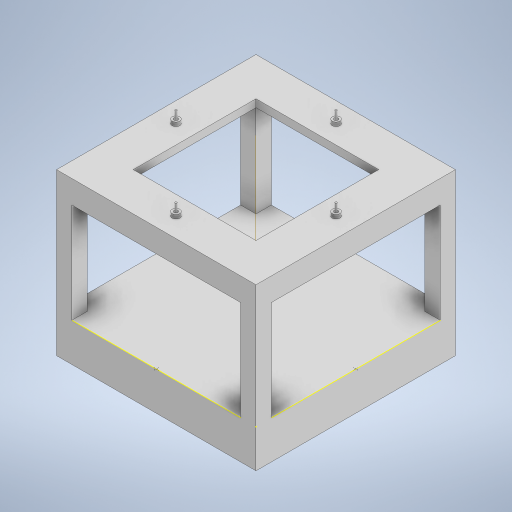
# Autodesk Inventor part: BaseMk1
Saved by Autodesk Inventor 2023 (Build 270158000, 158)
## iProperties
Created: 2023-03-23
Part Number: BaseMk1
Material: Generic
Document SubType Name: Modeling
Designer: czapa
Density: 1 g/cm^3
Appearance: Default
Author: czapa
Autodesk Inventor part; units mm, degrees
ref_plane "YZ Plane" through (0, 0, 0) normal (1, 0, 0) x (0, 1, 0)
ref_plane "XZ Plane" through (0, 0, 0) normal (0, 1, 0) x (-1, 0, 0)
sketch "Sketch1" plane through (0, 0, 0) normal (0, 1, 0) x (-1, 0, 0)
  line L0 (0, 0) -> (260, 0)
  line L1 (260, 0) -> (260, -260)
  line L2 (260, -260) -> (0, -260)
  line L3 (0, -260) -> (0, 0)
  dimension "d0" = 260
  dimension "d1" = 260
  constraints: 8 end point, 2 parallel, 1 horizontal, 1 perpendicular
  measures "d0" distance of L1.end L2.end
  measures "d1" distance of L0.end L1.end
extrude "Extrusion1" add sketch "Sketch1" along normal blind 200
sketch "Sketch2" plane through (0, 200, 0) normal (0, 1, 0) x (1, 0, 0)
  line L0 (-260, 0) -> (0, 0) projected
  line L1 (0, 0) -> (-20, 0)
  line L2 (-20, 0) -> (-20, 20)
  line L3 (-20, 20) -> (0, 20)
  line L4 (0, 20) -> (0, 0)
  line L5 (-260, 260) -> (-260, 0) projected
  line L6 (-260, 260) -> (-240, 260)
  line L7 (-240, 260) -> (-240, 240)
  line L8 (-240, 240) -> (-260, 240)
  line L9 (-260, 240) -> (-260, 260)
  line L10 (-240, 240) -> (-20, 240)
  line L11 (-20, 240) -> (-20, 20)
  line L12 (-20, 20) -> (-240, 20)
  line L13 (-240, 20) -> (-240, 240)
  dimension "d4" = 20
  dimension "d5" = 20
  dimension "d6" = 20
  dimension "d7" = 20
  constraints: 24 end point, 6 parallel, 3 horizontal, 3 perpendicular
  measures "d4" distance of L2.end L3.end
  measures "d5" distance of L1.end L2.end
  measures "d6" distance of L7.end L8.end
  measures "d7" distance of L6.end L7.end
sketch "Sketch3" plane through (-260, 0, 0) normal (0, 0, 1) x (1, 0, 0)
  line L0 (260, 200) -> (0, 200) projected
  line L1 (0, 200) -> (20, 200)
  line L2 (20, 200) -> (20, 180)
  line L3 (20, 180) -> (0, 180)
  line L4 (0, 180) -> (0, 200)
  line L5 (260, 0) -> (240, 0)
  line L6 (240, 0) -> (240, 50)
  line L7 (240, 50) -> (260, 50)
  line L8 (260, 50) -> (260, 0)
  line L9 (20, 180) -> (240, 180)
  line L10 (240, 180) -> (240, 50)
  line L11 (240, 50) -> (20, 50)
  line L12 (20, 50) -> (20, 180)
  dimension "d8" = 20
  dimension "d9" = 20
  dimension "d10" = 20
  dimension "d11" = 50
  constraints: 24 end point, 6 parallel, 3 horizontal, 3 perpendicular
  measures "d8" distance of L2.end L3.end
  measures "d9" distance of L1.end L2.end
  measures "d10" distance of L6.end L7.end
  measures "d11" distance of L5.end L6.end
extrude "Extrusion2" cut sketch "Sketch2" against normal blind 150 contours L12 L13 L10 L11
extrude "Extrusion3" cut sketch "Sketch3" against normal blind 260 contours L9 L10 L11 L12
ref_plane "Work Plane1" through (0, 0, -130) normal (0, 0, 1) x (1, 0, 0)
sketch "Sketch4" plane through (0, 0, 0) normal (1, 0, 0) x (0, 0, -1)
  line L0 (260, 200) -> (0, 200)
  line L1 (0, 200) -> (20, 200)
  line L2 (20, 200) -> (20, 180)
  line L3 (20, 180) -> (0, 180)
  line L4 (0, 180) -> (0, 200)
  line L5 (260, 0) -> (240, 0)
  line L6 (240, 0) -> (240, 50)
  line L7 (240, 50) -> (260, 50)
  line L8 (260, 50) -> (260, 0)
  line L9 (20, 180) -> (240, 180)
  line L10 (240, 180) -> (240, 50)
  line L11 (240, 50) -> (20, 50)
  line L12 (20, 50) -> (20, 180)
  point P0 (0, 0)
  dimension "d17" = 20
  dimension "d18" = 20
  dimension "d19" = 20
  dimension "d20" = 50
  constraints: 26 end point, 6 parallel, 3 horizontal, 3 perpendicular
  measures "d17" distance of L2.end L3.end
  measures "d18" distance of L1.end L2.end
  measures "d19" distance of L6.end L7.end
  measures "d20" distance of L5.end L6.end
extrude "Extrusion4" cut sketch "Sketch4" against normal blind 260 contours L9 L10 L11 L12
sketch "Sketch5" plane through (0, 200, 0) normal (0, 1, 0) x (1, 0, 0)
  line L0 (-260, 0) -> (0, 0) projected
  line L1 (-260, 260) -> (0, 260)
  line L2 (0, 260) -> (0, 0)
  line L3 (0, 0) -> (-260, 0)
  line L4 (-260, 0) -> (-260, 260)
  line L5 (-260, 260) -> (-210, 260)
  line L6 (-210, 260) -> (-210, 210)
  line L7 (-210, 210) -> (-260, 210)
  line L8 (-260, 210) -> (-260, 260)
  line L9 (0, 0) -> (-50, 0)
  line L10 (-50, 0) -> (-50, 50)
  line L11 (-50, 50) -> (0, 50)
  line L12 (0, 50) -> (0, 0)
  line L13 (-50, 50) -> (-210, 50)
  line L14 (-210, 50) -> (-210, 210)
  line L15 (-210, 210) -> (-50, 210)
  line L16 (-50, 210) -> (-50, 50)
  dimension "d23" = 50
  dimension "d24" = 50
  dimension "d25" = 50
  dimension "d26" = 50
  constraints: 32 end point, 8 parallel, 4 horizontal, 4 perpendicular
  measures "d23" distance of L6.end L7.end
  measures "d24" distance of L5.end L6.end
  measures "d25" distance of L10.end L11.end
  measures "d26" distance of L9.end L10.end
extrude "Extrusion5" add sketch "Sketch5" along normal blind 10 contours L4 L7 L14 L13 L10 L0 | L10 L11 L2 L0 | L4 L1 L6 L7 | L16 L15 L6 L1 L2 L11
sketch "Sketch6" plane through (0, 210, 0) normal (0, 1, 0) x (1, 0, 0)
  line L0 (0, 0) -> (-130, 0)
  line L1 (-130, 0) -> (-130, 130)
  line L2 (-130, 130) -> (0, 130)
  line L3 (0, 130) -> (0, 0)
  circle A0 centre (-130, 130) radius 97.5
  circle A1 centre (-130, 130) radius 111.25
  circle A2 centre (-130, 130) radius 104.375
  circle A3 centre (-25.625, 130) radius 1.25
  dimension "d33" = 208.75
  dimension "d29" = 130
  dimension "d30" = 130
  dimension "d31" = 195
  dimension "d32" = 222.5
  dimension "d43" = 2.5
  constraints: 8 end point, 3 centre point, 3 coincident, 2 parallel, 1 horizontal, 1 horizontal alignment, 1 perpendicular, 1 point on line, 2 other
  measures "d29" distance of L1.end L2.end
  measures "d30" distance of L0.end L1.end
  measures "d31" diameter of A0
  measures "d32" diameter of A1
  measures "d43" diameter of A3
sketch "Sketch7" plane through (0, 210, 0) normal (0, 1, 0) x (1, 0, 0)
  circle A0 centre (-25.625, 130) radius 2.5 projected
  circle A1 centre (-25.625, 130) radius 5
  point P0 (0, 0)
  dimension "d37" = 10
  constraints: 2 coincident, 1 centre point
  measures "d37" diameter of A1
extrude "Extrusion7" add sketch "Sketch7" along normal blind 5
sketch "Sketch8" plane through (0, 50, 0) normal (0, 1, 0) x (1, 0, 0)
  line L0 (-20, 0) -> (-240, 0) projected
  line L1 (0, 240) -> (0, 20) projected
  point P0 (0, 0)
  point P1 (-130, 0)
  point P2 (0, 130)
  point P3 (-130, 130)
  constraints: 2 midpoint
extrude "Extrusion8" add sketch "Sketch6" along normal blind 15 contours A3 A2 L2 | L2 A2 A3 | A2 L2 A3 | A3 L2 A2
pattern_circular "Circular Pattern2" count 4 over 360 about axis through (-130, 50, -130) along (0, 1, 0) of "Extrusion8", "Extrusion7"
body "Solid1"
